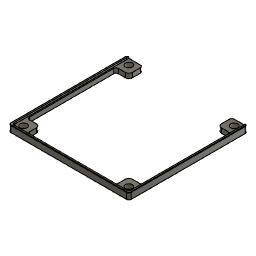
Diffuser (Autodesk Fusion 360 design; units mm, degrees)
Autodesk Fusion 360 part; units mm, degrees
note: some values were not read from the file. Set by a fixed rule: which sketch regions a step uses.
sketch "Sketch1" plane through (0, 0, 0) normal (0, 1, 0) x (1, 0, 0)
  line L0 (2, 0) -> (98.5, 0) construction
  line L1 (100.5, 2) -> (100.5, 98.5) construction
  line L2 (98.5, 100.5) -> (2, 100.5) construction
  line L3 (0, 98.5) -> (0, 2) construction
  circle A0 centre (5, 95.5) radius 1.6 construction
  circle A1 centre (95.5, 95.5) radius 1.6 construction
  circle A2 centre (5, 5) radius 1.6 construction
  circle A3 centre (95.5, 5) radius 1.6 construction
  line L4 (99.5, 97.5) -> (99.5, 3)
  line L5 (97.5, 1) -> (3, 1)
  line L6 (1, 3) -> (1, 97.5)
  line L7 (102, 98.5) -> (102, 0.5)
  line L8 (100, -1.5) -> (0.5, -1.5)
  line L9 (-1.5, 0.5) -> (-1.5, 98.5)
  arc A4 (100, -1.5) -> (102, 0.5) centre (100, 0.5) ccw
  arc A5 (-1.5, 0.5) -> (0.5, -1.5) centre (0.5, 0.5) ccw
  arc A6 (0.5, 100.5) -> (-1.5, 98.5) centre (0.5, 98.5) ccw
  arc A7 (102, 98.5) -> (100, 100.5) centre (100, 98.5) ccw
  arc A8 (97.5, 1) -> (99.5, 3) centre (97.5, 3) ccw
  arc A9 (99.5, 97.5) -> (97.5, 99.5) centre (97.5, 97.5) ccw
  arc A10 (3, 99.5) -> (1, 97.5) centre (3, 97.5) ccw
  arc A11 (1, 3) -> (3, 1) centre (3, 3) ccw
  line L10 (99.5, 88.5) -> (91.5, 88.5)
  line L11 (88.5, 91.5) -> (88.5, 99.5)
  line L12 (99.5, 12) -> (91.5, 12)
  line L13 (88.5, 9) -> (88.5, 1)
  line L14 (1, 12) -> (9, 12)
  line L15 (12, 9) -> (12, 1)
  line L16 (12, 99.5) -> (12, 91.5)
  line L17 (9, 88.5) -> (1, 88.5)
  arc A12 (88.5, 91.5) -> (91.5, 88.5) centre (91.5, 91.5) ccw
  arc A13 (9, 88.5) -> (12, 91.5) centre (9, 91.5) ccw
  arc A14 (12, 9) -> (9, 12) centre (9, 9) ccw
  arc A15 (91.5, 12) -> (88.5, 9) centre (91.5, 9) ccw
  circle A16 centre (95.5, 95.5) radius 3
  circle A17 centre (95.5, 5) radius 3
  circle A18 centre (5, 5) radius 3
  circle A19 centre (5, 95.5) radius 3
  line L18 (3, 99.5) -> (12, 99.5)
  line L19 (88.5, 99.5) -> (97.5, 99.5)
  line L20 (88.5, 99.5) -> (88.5, 100.5)
  line L21 (12, 99.5) -> (12, 100.5)
  line L22 (0.5, 100.5) -> (12, 100.5)
  line L23 (88.5, 100.5) -> (100, 100.5)
  arc A20 (98.5, 0) -> (100.5, 2) centre (98.5, 2) ccw construction
  arc A21 (100.5, 98.5) -> (98.5, 100.5) centre (98.5, 98.5) ccw construction
  arc A22 (2, 100.5) -> (0, 98.5) centre (2, 98.5) ccw construction
  arc A23 (0, 2) -> (2, 0) centre (2, 2) ccw construction
  point P0 (100.5, 0)
  point P1 (0, 100.5)
  dimension "d1" = 100.5
  dimension "d2" = 100.5
  dimension "d3" = 3.2
  dimension "d4" = 5
  dimension "d5" = 5
  dimension "d6" = 3.2
  dimension "d7" = 3.2
  dimension "d8" = 3.2
  dimension "d9" = 5
  dimension "d10" = 1
  dimension "d11" = 1
  dimension "d12" = 1
  dimension "d13" = 1
  dimension "d14" = 2.5
  dimension "d15" = 2.5
  dimension "d16" = 2.5
  dimension "d17" = 2
  dimension "d18" = 2
  dimension "d19" = 2
  dimension "d20" = 2
  dimension "d21" = 2
  dimension "d22" = 2
  dimension "d23" = 2
  dimension "d24" = 2
  dimension "d27" = 12
  dimension "d28" = 12
  dimension "d29" = 12
  dimension "d30" = 12
  dimension "d31" = 12
  dimension "d32" = 12
  dimension "d33" = 12
  dimension "d34" = 12
  dimension "d35" = 3
  dimension "d36" = 3
  dimension "d37" = 6
  dimension "d38" = 6
  dimension "d39" = 6
  dimension "d40" = 6
  dimension "d43" = 2
  dimension "d44" = 2
  dimension "d45" = 2
  dimension "d46" = 2
  constraint horizontal L0
  constraint vertical L1
  constraint horizontal L2
  constraint vertical L3
  constraint horizontal A0.centre A1.centre
  constraint vertical A0.centre A2.centre
  constraint vertical A1.centre A3.centre
  constraint horizontal A2.centre A3.centre
  constraint horizontal L18
  constraint vertical L4
  constraint horizontal L5
  constraint vertical L6
  constraint horizontal L22
  constraint vertical L7
  constraint horizontal L8
  constraint vertical L9
  constraint collinear L2 L22
  constraint tangent L7 A4
  constraint tangent L8 A4
  constraint tangent L8 A5
  constraint tangent L9 A5
  constraint tangent A6 L22
  constraint tangent L9 A6
  constraint tangent A7 L22
  constraint tangent L7 A7
  constraint tangent L4 A8
  constraint tangent L5 A8
  constraint tangent A9 L18
  constraint tangent L4 A9
  constraint tangent A10 L18
  constraint tangent L6 A10
  constraint tangent L5 A11
  constraint tangent L6 A11
  constraint coincident L4 L10.start
  constraint perpendicular L4 L10
  constraint coincident L11.end L18
  constraint perpendicular L11 L18
  constraint coincident L4 L12.start
  constraint perpendicular L4 L12
  constraint coincident L5 L13.end
  constraint perpendicular L5 L13
  constraint coincident L6 L14.start
  constraint perpendicular L6 L14
  constraint coincident L5 L15.end
  constraint perpendicular L5 L15
  constraint perpendicular L16 L18
  constraint coincident L6 L17.end
  constraint perpendicular L6 L17
  constraint tangent L10 A12
  constraint tangent L11 A12
  constraint tangent L16 A13
  constraint tangent L17 A13
  constraint equal A12 A13
  constraint tangent L14 A14
  constraint tangent L15 A14
  constraint equal A12 A14
  constraint tangent L12 A15
  constraint tangent L13 A15
  constraint concentric A1 A16
  constraint concentric A3 A17
  constraint concentric A2 A18
  constraint concentric A0 A19
  constraint collinear L18 L19
  constraint coincident L2 L20.end
  constraint coincident L2 L21.end
  constraint collinear L22 L23
  constraint coincident P0 L0
  constraint coincident P0 L1
  constraint tangent L0 A20
  constraint tangent L1 A20
  constraint tangent L1 A21
  constraint tangent L2 A21
  constraint coincident P1 L2
  constraint coincident P1 L3
  constraint tangent L2 A22
  constraint tangent L3 A22
  constraint coincident origin L0
  constraint coincident origin L3
  constraint tangent L0 A23
  constraint tangent L3 A23
  measures "d1" distance of origin P0
  measures "d2" distance of origin P1
  measures "d3" diameter of A0
  measures "d4" distance of L3 A0.centre
  measures "d5" distance of L2 A0.centre
  measures "d6" diameter of A1
  measures "d7" diameter of A2
  measures "d8" diameter of A3
  measures "d9" distance of L1 A1.centre
  measures "d10" distance of L2 L18
  measures "d11" distance of L1 L4
  measures "d12" distance of L0 L5
  measures "d13" distance of L3 L6
  measures "d14" distance of L4 L7
  measures "d15" distance of L5 L8
  measures "d16" distance of L6 L9
  measures "d17" radius of A4
  measures "d18" radius of A5
  measures "d19" radius of A6
  measures "d20" radius of A7
  measures "d21" radius of A8
  measures "d22" radius of A9
  measures "d23" radius of A10
  measures "d24" radius of A11
  measures "d27" distance of L10 L22
  measures "d28" distance of L1 L11
  measures "d29" distance of L1 L13
  measures "d30" distance of L0 L12
  measures "d31" distance of L3 L15
  measures "d32" distance of L0 L14
  measures "d33" distance of L2 L17
  measures "d34" distance of L3 L16
  measures "d35" radius of A12
  measures "d36" radius of A15
  measures "d37" diameter of A16
  measures "d38" diameter of A17
  measures "d39" diameter of A18
  measures "d40" diameter of A19
  measures "d43" radius of A20
  measures "d44" radius of A21
  measures "d45" radius of A22
  measures "d46" radius of A23
extrude "Extrude1" add sketch "Sketch1" along normal blind 4
sketch "Sketch2" plane through (0, 4, 0) normal (0, 1, 0) x (-1, 0, 0)
  circle A0 centre (-95.5, -5) radius 3
  circle A1 centre (-5, -5) radius 3
  circle A2 centre (-95.5, -95.5) radius 3
  circle A3 centre (-5, -95.5) radius 3
  arc A4 (-88.5, -91.5) -> (-91.5, -88.5) centre (-91.5, -91.5) ccw
  line L0 (-91.5, -88.5) -> (-99.5, -88.5)
  line L1 (-99.5, -88.5) -> (-99.5, -12)
  line L2 (-99.5, -12) -> (-91.5, -12)
  arc A5 (-91.5, -12) -> (-88.5, -9) centre (-91.5, -9) ccw
  line L3 (-88.5, -9) -> (-88.5, -1)
  line L4 (-88.5, -1) -> (-12, -1)
  line L5 (-12, -1) -> (-12, -9)
  arc A6 (-12, -9) -> (-9, -12) centre (-9, -9) ccw
  line L6 (-9, -12) -> (-1, -12)
  line L7 (-1, -12) -> (-1, -88.5)
  line L8 (-1, -88.5) -> (-9, -88.5)
  arc A7 (-9, -88.5) -> (-12, -91.5) centre (-9, -91.5) ccw
  line L9 (-12, -91.5) -> (-12, -100.5)
  line L10 (-12, -100.5) -> (-0.5, -100.5)
  arc A8 (-0.5, -100.5) -> (1.5, -98.5) centre (-0.5, -98.5) ccw
  line L11 (1.5, -98.5) -> (1.5, -0.5)
  arc A9 (1.5, -0.5) -> (-0.5, 1.5) centre (-0.5, -0.5) ccw
  line L12 (-0.5, 1.5) -> (-100, 1.5)
  arc A10 (-100, 1.5) -> (-102, -0.5) centre (-100, -0.5) ccw
  line L13 (-102, -0.5) -> (-102, -98.5)
  arc A11 (-102, -98.5) -> (-100, -100.5) centre (-100, -98.5) ccw
  line L14 (-100, -100.5) -> (-88.5, -100.5)
  line L15 (-88.5, -100.5) -> (-88.5, -91.5)
  arc A12 (0, -2) -> (-2, 0) centre (-2, -2) ccw
  line L16 (-2, 0) -> (-98.5, 0)
  arc A13 (1.5, -0.5) -> (-0.5, 1.5) centre (-0.5, -0.5) ccw
  line L17 (-0.5, 1.5) -> (-100, 1.5)
  arc A14 (-98.5, 0) -> (-100.5, -2) centre (-98.5, -2) ccw
  line L18 (-100.5, -2) -> (-100.5, -98.5)
  arc A15 (-100, 1.5) -> (-102, -0.5) centre (-100, -0.5) ccw
  line L19 (-102, -98.5) -> (-102, -0.5)
  line L20 (-98.5, -100.5) -> (-2, -100.5)
  line L21 (-100, -100.5) -> (-88.5, -100.5)
  arc A16 (-102, -98.5) -> (-100, -100.5) centre (-100, -98.5) ccw
  line L22 (-102, -0.5) -> (-102, -98.5)
  line L23 (0, -98.5) -> (0, -2)
  arc A17 (-0.5, -100.5) -> (1.5, -98.5) centre (-0.5, -98.5) ccw
  line L24 (1.5, -98.5) -> (1.5, -0.5)
  line L25 (0, -98.5) -> (0, -100.5)
  line L26 (-100.5, -98.5) -> (-100.5, -100.5)
  constraint coincident L23.start L25.start
  constraint coincident L10 L25.end
  constraint perpendicular L10 L25
  constraint coincident L18.end L26.start
  constraint coincident L21 L26.end
  constraint perpendicular L21 L26
extrude "Extrude3" add sketch "Sketch2" along normal blind 1.5 contours A8 L11 A9 L12 A10 L13 A11 A12 L16 A13 L17 A14 L18 A15 L19 A16 L22 L23 A17 L24 L25 L26
fillet "Fillet2" radius 0.3 7 edges at (-1.0811, 5.5, -99.7247) (-1.5, 5.5, -49.5) (-0.9142, 5.5, 0.9142) (50.25, 5.5, 1.5) (101.4142, 5.5, 0.9142) (102, 5.5, -49.5) (101.5811, 5.5, -99.7247)
extrude "Extrude2" add sketch "Sketch2" along normal blind 1.5 contours A8 L11 A9 L12 A10 L13 A11 A12 L16 A13 L17 A14 L18 A15 L19 A16 L22 L23 A17 L24 L25 L26
fillet "Fillet1" radius 0.3 7 edges at (-1.0811, 5.5, -99.7247) (-1.5, 5.5, -49.5) (-0.9142, 5.5, 0.9142) (50.25, 5.5, 1.5) (101.4142, 5.5, 0.9142) (102, 5.5, -49.5) (101.5811, 5.5, -99.7247)
fillet "Fillet3" radius 2 1 edges at (12, 2, -100.5)
fillet "Fillet3" radius 2 1 edges at (88.5, 2, -100.5)
fillet "Fillet3" radius 2 1 edges at (99.5, 2, -88.5)
fillet "Fillet3" radius 2 1 edges at (99.5, 2, -12)
fillet "Fillet3" radius 2 1 edges at (88.5, 2, -1)
fillet "Fillet3" radius 2 1 edges at (12, 2, -1)
fillet "Fillet3" radius 2 1 edges at (1, 2, -12)
fillet "Fillet3" radius 2 1 edges at (1, 2, -88.5)
